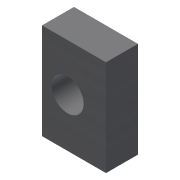
# Autodesk Inventor part: box
Saved by Autodesk Inventor 2022 Beta2 (Build 260130000, 130) ContinuousBuild 0
## iProperties
Shininess: 64.0
Length Units: 11269
Angle Units: 11279
Time Units: 11290
Mass Units: 11283
Length Display Precision: 3
Angle Display Precision: 2
Created: 2001-12-18
Part Number: box
Document SubType Name: Modeling
Designer: Administrator
Density: 1 g/cm^3
Material: Generic
Appearance: Light Gray
Density: 0.0
Volumn: 0.0
Area: 0.0
PropertySet Name: Model Information
Control State: 0
Master: False
Checked Out: False
Author: Administrator
Autodesk Inventor part; units mm, degrees
ref_plane "YZ Plane" through (0, 0, 0) normal (1, 0, 0) x (0, 1, 0)
ref_plane "XZ Plane" through (0, 0, 0) normal (0, 1, 0) x (-1, 0, 0)
ref_plane "XY Plane" through (0, 0, 0) normal (0, 0, 1) x (1, 0, 0)
sketch "Sketch1" plane through (0, 0, 0) normal (0, 0, 1) x (1, 0, 0)
  line L0 (-19.1729, 62.3255) -> (30.8271, 62.3255)
  line L1 (30.8271, 62.3255) -> (30.8271, -12.6745)
  line L2 (30.8271, -12.6745) -> (-19.1729, -12.6745)
  line L3 (-19.1729, -12.6745) -> (-19.1729, 62.3255)
  dimension "d0" = 50
  dimension "d1" = 75
  constraints: 8 end point, 2 parallel, 1 horizontal, 1 perpendicular
  measures "d0" distance of L1.end L2.end
  measures "d1" distance of L2.end L0.start
extrude "Extrusion1" add sketch "Sketch1" along normal blind 25
sketch "Sketch2" plane through (0, 0, 25) normal (0, 0, 1) x (1, 0, 0)
  circle A0 centre (0.8271, 25.3255) radius 12.5
  point P0 (-19.1729, -12.6745)
  dimension "d4" = 20
  dimension "d5" = 25
  dimension "d8" = 38
  constraints: 1 centre point
  measures "d4" horizontal distance of point (-19.173, -12.675) A0.centre
  measures "d5" diameter of A0
  measures "d8" vertical distance of A0.centre point (-19.173, -12.675)
extrude "Extrusion2" cut sketch "Sketch2" against normal up to surface (25 mm away)
body "Solid1"
